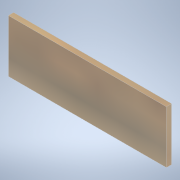
# Autodesk Inventor part: Eyebrow1
Saved by Autodesk Inventor 2021 (Build 250183000, 183)
## iProperties
Created: 2023-05-31
Part Number: Eyebrow1
Material: Wood (Maple)
Document SubType Name: Modeling
Designer: shrus
Density: 0.67 g/cm^3
Appearance: Natural Maple - Glossy Dark Tint
Author: shrus
Autodesk Inventor part; units mm, degrees
ref_plane "YZ Plane" through (0, 0, 0) normal (1, 0, 0) x (0, 1, 0)
ref_plane "XZ Plane" through (0, 0, 0) normal (0, 1, 0) x (-1, 0, 0)
ref_plane "XY Plane" through (0, 0, 0) normal (0, 0, 1) x (1, 0, 0)
sketch "Sketch1" plane through (0, 0, 0) normal (0, 0, 1) x (1, 0, 0)
  line L0 (-13.5457, 10.79) -> (16.4543, 10.79)
  line L1 (16.4543, 10.79) -> (16.4543, 0.79)
  line L2 (16.4543, 0.79) -> (-13.5457, 0.79)
  line L3 (-13.5457, 0.79) -> (-13.5457, 10.79)
  point P0 (0, 0)
  dimension "d0" = 30
  dimension "d1" = 10
  constraints: 8 end point, 2 horizontal, 2 perpendicular
  measures "d0" distance of L0.start L0.end
  measures "d1" distance of L0.end L1.end
extrude "Extrusion1" add sketch "Sketch1" along normal blind 1
body "Solid1"
